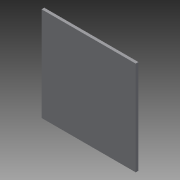
# Autodesk Inventor part: fai20_sikiita
Saved by Autodesk Inventor 2013 (Build 170138000, 138)
## iProperties
Created: 2014-04-21
Part Number: fai20_sikiita
Material: 一般
Document SubType Name: Modeling
Designer: andou
Density: 1 g/cm^3
Author: andou
Autodesk Inventor part; units mm, degrees
ref_plane "YZ Plane" through (0, 0, 0) normal (1, 0, 0) x (0, 1, 0)
ref_plane "XZ Plane" through (0, 0, 0) normal (0, 1, 0) x (-1, 0, 0)
ref_plane "XY Plane" through (0, 0, 0) normal (0, 0, 1) x (1, 0, 0)
sketch "スケッチ1" plane through (0, 0, 0) normal (0, 1, 0) x (-1, 0, 0)
  line L0 (-52, 52) -> (52, 52)
  line L1 (52, 52) -> (52, -52)
  line L2 (52, -52) -> (-52, -52)
  line L3 (-52, -52) -> (-52, 52)
  point P0 (0, 0)
  dimension "d0" = 104
  dimension "d2" = 104
  dimension "d3" = 52
  dimension "d4" = 52
  constraints: 8 end point, 2 parallel, 1 horizontal, 1 perpendicular
  measures "d0" distance of L0.start L0.end
  measures "d2" distance of L2.end L0.start
  measures "d3" distance from line of L0 point (0, 0)
  measures "d4" distance from line of L3 point (0, 0)
extrude "押し出し1" add sketch "スケッチ1" along normal blind 2
sketch "スケッチ2" plane through (0, 2, 0) normal (0, 1, 0) x (1, 0, 0)
  line L0 (-52, -52) -> (52, -52) projected
  line L1 (52, -52) -> (52, 52) projected
  line L2 (52, 52) -> (-52, 52) projected
  line L3 (-52, 52) -> (-52, -52) projected
  circle A0 centre (-42, -42) radius 10
  circle A1 centre (-14, -42) radius 10
  circle A2 centre (14, -42) radius 10
  circle A3 centre (-42, -14) radius 10
  circle A4 centre (-14, -14) radius 10
  circle A5 centre (14, -14) radius 10
  circle A6 centre (-42, 14) radius 10
  circle A7 centre (-14, 14) radius 10
  circle A8 centre (14, 14) radius 10
  circle A9 centre (42, -42) radius 10
  circle A10 centre (42, -14) radius 10
  circle A11 centre (42, 14) radius 10
  circle A12 centre (42, 42) radius 10
  circle A13 centre (14, 42) radius 10
  circle A14 centre (-14, 42) radius 10
  circle A15 centre (-42, 42) radius 10
  point P0 (0, 0)
  dimension "d7" = 20
  dimension "d43" = 28
  dimension "d44" = 28
  dimension "d45" = 28
  dimension "d46" = 10
  dimension "d47" = 10
  dimension "d48" = 10
  dimension "d49" = 10
  dimension "d50" = 10
  dimension "d51" = 10
  dimension "d52" = 28
  dimension "d53" = 28
  dimension "d54" = 28
  dimension "d55" = 28
  dimension "d56" = 28
  dimension "d57" = 28
  dimension "d58" = 28
  dimension "d59" = 28
  dimension "d60" = 28
  dimension "d61" = 28
  dimension "d62" = 28
  dimension "d63" = 10
  dimension "d64" = 10
  dimension "d65" = 28
  dimension "d66" = 28
  dimension "d67" = 28
  dimension "d68" = 28
  dimension "d69" = 28
  dimension "d70" = 28
  dimension "d71" = 28
  dimension "d72" = 28
  dimension "d73" = 28
  dimension "d74" = 28
  constraints: 16 centre point, 15 equal radius
  measures "d7" diameter of A0
  measures "d43" distance of A1.centre A0.centre
  measures "d44" distance of A2.centre A1.centre
  measures "d45" distance of A9.centre A2.centre
  measures "d46" distance from line of A0.centre L0
  measures "d47" distance from line of A1.centre L0
  measures "d48" distance from line of L0 A2.centre
  measures "d49" distance from line of A9.centre L0
  measures "d50" distance from line of A0.centre L3
  measures "d51" distance from line of A3.centre L3
  measures "d52" distance of A4.centre A3.centre
  measures "d53" distance of A5.centre A4.centre
  measures "d54" distance of A10.centre A5.centre
  measures "d55" distance of A10.centre A9.centre
  measures "d56" distance of A5.centre A2.centre
  measures "d57" distance of A4.centre A1.centre
  measures "d58" distance of A3.centre A0.centre
  measures "d59" distance of A6.centre A3.centre
  measures "d60" distance of A15.centre A6.centre
  measures "d61" distance of A4.centre A7.centre
  measures "d62" distance of A14.centre A7.centre
  measures "d63" distance from line of L3 A6.centre
  measures "d64" distance from line of L3 A15.centre
  measures "d65" distance of A14.centre A15.centre
  measures "d66" distance of A6.centre A7.centre
  measures "d67" distance of A8.centre A7.centre
  measures "d68" distance of A8.centre A11.centre
  measures "d69" distance of A5.centre A8.centre
  measures "d70" distance of A11.centre A10.centre
  measures "d71" distance of A11.centre A12.centre
  measures "d72" distance of A8.centre A13.centre
  measures "d73" distance of A13.centre A14.centre
  measures "d74" distance of A12.centre A13.centre
extrude "押し出し2" add sketch "スケッチ2" along normal blind 1 contours L3 A0 L0 | A0 L3 A15 L2 A12 L1 A9 L0 | A9 L1 L0 | L3 L2 A15 | A12 L2 L1
